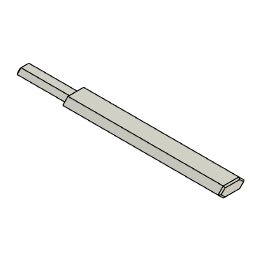
Tibia foot v11 (Autodesk Fusion 360 design; units mm, degrees)
Autodesk Fusion 360 part; units mm, degrees
sketch "Sketch1" plane through (0, 0, 0) normal (1, 0, 0) x (0, 1, 0)
  line L0 (-3, 2) -> (3, 2)
  line L1 (3, 2) -> (3, -2)
  line L2 (3, -2) -> (-3, -2)
  line L3 (-3, -2) -> (-3, 2)
  line L4 (3, 2) -> (5, 0)
  line L5 (5, 0) -> (3, -2)
  line L6 (-3, 2) -> (-5, 0)
  line L7 (-5, 0) -> (-3, -2)
  line L8 (-3, 2) -> (3, -2) construction
  line L9 (3, 2) -> (-3, -2) construction
  dimension "d1" = 10
  dimension "d2" = 2
  dimension "d3" = 4
  constraint horizontal L0
  constraint vertical L1
  constraint horizontal L2
  constraint vertical L3
  constraint equal L4 L5
  constraint equal L6 L7
  constraint equal L4 L6
  constraint coincident origin L9
  constraint coincident origin L8
  measures "d1" distance of L4.end L6.end
  measures "d2" distance of L1 L4.end
  measures "d3" distance of L0 L2
extrude "Extrude1" add sketch "Sketch1" along normal blind 60
sketch "Sketch2" plane through (0, 0, 0) normal (-1, 0, 0) x (0, -1, 0)
  line L0 (5, 0) -> (3, 2)
  line L1 (-3, 2) -> (-5, 0)
  line L2 (-5, 0) -> (-3, -2)
  line L3 (3, -2) -> (5, 0)
  line L4 (-1.5, 1) -> (1.5, 1)
  line L5 (1.5, 1) -> (1.5, -2)
  line L6 (1.5, -2) -> (-1.5, -2)
  line L7 (-1.5, -2) -> (-1.5, 1)
  line L8 (1.5, 1) -> (3, -0.5)
  line L9 (3, -0.5) -> (1.5, -2)
  line L10 (-1.5, 1) -> (-3, -0.5)
  line L11 (-3, -0.5) -> (-1.5, -2)
  line L12 (3, 2) -> (-3, 2)
  dimension "d12" = 3
  dimension "d13" = 1.5
  dimension "d14" = 45
  dimension "d15" = 45
  dimension "d16" = 1
  constraint horizontal L4
  constraint vertical L5
  constraint horizontal L6
  constraint vertical L7
  constraint equal L4 L5
  constraint equal L8 L9
  constraint equal L10 L11
  measures "d12" distance of L4.start L4.end
  measures "d13" distance of origin L5
  measures "d14" angle of L5 L8
  measures "d15" angle of L7 L10
  measures "d16" distance of L4 L12
extrude "Extrude2" add sketch "Sketch2" along normal blind 20
chamfer "Chamfer1" distance 0.5 angle 45 1 faces at (60, -1, -0.6667)
chamfer "Chamfer3" distance 0.5 angle 45 1 faces at (-20, 0.5, 0)
equation "d13 = d12 / 2"
